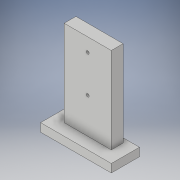
# Autodesk Inventor part: Frame
Saved by Autodesk Inventor 2017 (Build 210142000, 142)
## iProperties
Created: 2018-03-04
Part Number: Frame
Material: Generic
Document SubType Name: Modeling
Designer: Russ
Density: 1 g/cm^3
Appearance: Default
Author: Russ
Autodesk Inventor part; units mm, degrees
ref_plane "YZ Plane" through (0, 0, 0) normal (1, 0, 0) x (0, 1, 0)
ref_plane "XZ Plane" through (0, 0, 0) normal (0, 1, 0) x (-1, 0, 0)
ref_plane "XY Plane" through (0, 0, 0) normal (0, 0, 1) x (1, 0, 0)
sketch "Sketch1" plane through (0, 0, 0) normal (0, 0, 1) x (1, 0, 0)
  circle A0 centre (0, 0) radius 7.62
  circle A1 centre (0, -40.005) radius 30.48
  circle A2 centre (0, 0) radius 1.55
  circle A3 centre (0, -40.005) radius 1.55
  line L0 (-25.4, 14.478) -> (25.4, 14.478)
  line L1 (25.4, 14.478) -> (25.4, -87.122)
  line L2 (25.4, -87.122) -> (-25.4, -87.122)
  line L3 (-25.4, -87.122) -> (-25.4, 14.478)
  line L4 (-25.4, -87.122) -> (-38.1, -87.122)
  line L5 (-38.1, -87.122) -> (-38.1, -78.232)
  line L6 (-38.1, -78.232) -> (-25.4, -78.232)
  line L7 (25.4, -87.122) -> (38.1, -87.122)
  line L8 (38.1, -87.122) -> (38.1, -78.232)
  line L9 (38.1, -78.232) -> (25.4, -78.232)
  dimension "d0" = 40.005
  dimension "d1" = 15.24
  dimension "d2" = 60.96
  dimension "d3" = 3.1
  dimension "d4" = 3.1
  dimension "d5" = 14.478
  dimension "d6" = 25.4
  dimension "d7" = 25.4
  dimension "d8" = 101.6
  dimension "d9" = 12.7
  dimension "d10" = 12.7
  dimension "d11" = 8.89
  constraints: 20 end point, 5 point on line, 4 centre point, 4 perpendicular, 3 coincident, 2 horizontal, 2 parallel
  measures "d0" distance of A1.centre point (0, 0)
  measures "d1" diameter of A0
  measures "d2" diameter of A1
  measures "d3" diameter of A2
  measures "d4" diameter of A3
  measures "d5" distance from line of L0 point (0, 0)
  measures "d6" distance from line of point (0, 0) L1
  measures "d7" distance from line of A2.centre L3
  measures "d8" distance of L0.end L1.end
  measures "d9" distance between parallel lines of L8 L1
  measures "d10" distance between parallel lines of L3 L5
  measures "d11" distance of L4.end L5.end
extrude "Extrusion1" add sketch "Sketch1" along normal blind 12.7 contours A0 | L1 A1 L3 | A1 L3 L0 L1 | L1 L2 L3 A1 | L9 L8 L7 L1 | L3 L4 L5 L6
sketch "Sketch3" plane through (0, 0, 12.7) normal (0, 0, 1) x (1, 0, 0)
  line L0 (-25.4, -78.232) -> (-38.1, -78.232) projected
  line L1 (38.1, -87.122) -> (38.1, -78.232) projected
  line L2 (-38.1, -78.232) -> (38.1, -78.232)
  line L3 (38.1, -78.232) -> (38.1, -87.122)
  line L4 (38.1, -87.122) -> (-38.1, -87.122)
  line L5 (-38.1, -87.122) -> (-38.1, -78.232)
  point P0 (0, 0)
  constraints: 8 end point, 2 parallel, 1 horizontal, 1 perpendicular
extrude "Extrusion3" add sketch "Sketch3" along normal blind 12.7
sketch "Sketch5" plane through (0, 0, 0) normal (0, 0, -1) x (-1, 0, 0)
  line L0 (38.1, -87.122) -> (-38.1, -87.122) projected
  line L1 (38.1, -78.232) -> (38.1, -87.122) projected
  line L2 (-38.1, -87.122) -> (38.1, -87.122)
  line L3 (38.1, -87.122) -> (38.1, -78.232)
  line L4 (38.1, -78.232) -> (-38.1, -78.232)
  line L5 (-38.1, -78.232) -> (-38.1, -87.122)
  point P0 (0, 0)
  constraints: 8 end point, 2 parallel, 1 horizontal, 1 perpendicular
extrude "Extrusion4" add sketch "Sketch5" along normal blind 4.9022
body "Solid1"
